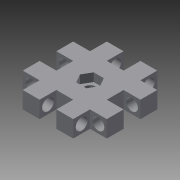
# Autodesk Inventor part: crossCenterMini
Saved by Autodesk Inventor 2015 (Build 190159000, 159)
## iProperties
Created: 2016-10-15
Part Number: crossCenterMini
Material: Generic
Document SubType Name: Modeling
Designer: Bardo91
Density: 1 g/cm^3
Appearance: Default
Author: Bardo91
Autodesk Inventor part; units mm, degrees
ref_plane "YZ Plane" through (0, 0, 0) normal (1, 0, 0) x (0, 1, 0)
ref_plane "XZ Plane" through (0, 0, 0) normal (0, 1, 0) x (-1, 0, 0)
ref_plane "XY Plane" through (0, 0, 0) normal (0, 0, 1) x (1, 0, 0)
sketch "Sketch1" plane through (0, 0, 0) normal (0, 0, 1) x (1, 0, 0)
  line L0 (0, 0) -> (0, 5)
  line L1 (0, 5) -> (5, 5)
  line L2 (5, 5) -> (5, 0)
  line L3 (5, 0) -> (10, 0)
  line L4 (10, 0) -> (10, 5)
  line L5 (10, 5) -> (15, 5)
  line L6 (15, 5) -> (15, 0)
  line L7 (15, 0) -> (20, 0)
  line L8 (20, 0) -> (20, -5)
  line L9 (20, -5) -> (15, -5)
  line L10 (15, -5) -> (15, -10)
  line L11 (15, -10) -> (20, -10)
  line L12 (20, -10) -> (20, -15)
  line L13 (20, -15) -> (15, -15)
  line L14 (15, -15) -> (15, -20)
  line L15 (15, -20) -> (10, -20)
  line L16 (10, -20) -> (10, -15)
  line L17 (10, -15) -> (5, -15)
  line L18 (5, -15) -> (5, -20)
  line L19 (5, -20) -> (0, -20)
  line L20 (0, -20) -> (0, -15)
  line L21 (0, -15) -> (-5, -15)
  line L22 (-5, -15) -> (-5, -10)
  line L23 (-5, -10) -> (0, -10)
  line L24 (0, -10) -> (0, -5)
  line L25 (0, -5) -> (-5, -5)
  line L26 (-5, -5) -> (-5, 0)
  line L27 (-5, 0) -> (0, 0)
  dimension "d0" = 5
  dimension "d1" = 5
  dimension "d2" = 5
  dimension "d3" = 5
  dimension "d4" = 5
  dimension "d5" = 5
  dimension "d6" = 5
  dimension "d7" = 5
  dimension "d8" = 5
  dimension "d9" = 5
  dimension "d10" = 5
  dimension "d11" = 5
  dimension "d12" = 5
  dimension "d13" = 5
  dimension "d14" = 5
  dimension "d15" = 5
  dimension "d16" = 5
  dimension "d17" = 5
  dimension "d18" = 5
  dimension "d19" = 5
  dimension "d20" = 5
  dimension "d21" = 5
  dimension "d22" = 5
  dimension "d23" = 5
  dimension "d24" = 5
  dimension "d25" = 90
  dimension "d26" = 5
  dimension "d27" = 5
  constraints: 56 end point, 16 point on line, 10 perpendicular, 2 vertical
  measures "d0" distance of L0.start L0.end
  measures "d1" distance of L0.end L1.end
  measures "d2" distance of L1.end L2.end
  measures "d3" distance of L2.end L3.end
  measures "d4" distance of L3.end L4.end
  measures "d5" distance of L4.end L5.end
  measures "d6" distance of L5.end L6.end
  measures "d7" distance of L6.end L7.end
  measures "d8" distance of L7.end L8.end
  measures "d9" distance of L8.end L9.end
  measures "d10" distance of L9.end L10.end
  measures "d11" distance of L10.end L11.end
  measures "d12" distance of L11.end L12.end
  measures "d13" distance of L12.end L13.end
  measures "d14" distance of L13.end L14.end
  measures "d15" distance of L14.end L15.end
  measures "d16" distance of L15.end L16.end
  measures "d17" distance of L16.end L17.end
  measures "d18" distance of L17.end L18.end
  measures "d19" distance of L18.end L19.end
  measures "d20" distance of L19.end L20.end
  measures "d21" distance of L20.end L21.end
  measures "d22" distance of L21.end L22.end
  measures "d23" distance of L22.end L23.end
  measures "d24" distance of L23.end L24.end
  measures "d25" angle of L24 L23
  measures "d26" distance of L24.end L25.end
  measures "d27" distance of L25.end L26.end
extrude "Extrusion1" add sketch "Sketch1" along normal blind 5
sketch "Sketch2" plane through (0, 0, 5) normal (0, 0, 1) x (1, 0, 0)
  line L0 (15, -10) -> (15, -5) projected
  line L1 (15, -7.5) -> (0, -7.5)
  line L2 (0, -10) -> (0, -5) projected
  circle A0 centre (7.5, -7.5) radius 1.75
  point P0 (0, 0)
  dimension "d30" = 3.5
  constraints: 3 midpoint, 2 end point, 1 centre point
  measures "d30" diameter of A0
extrude "Extrusion2" cut sketch "Sketch2" against normal blind 5
sketch "Sketch3" plane through (0, 0, 5) normal (0, 0, 1) x (1, 0, 0)
  circle A0 centre (7.5, -7.5) radius 1.75 projected
  line L0 (7.5, -7.5) -> (10.5, -7.5)
  line L1 (10.5, -7.5) -> (9, -4.9019)
  line L2 (7.5, -7.5) -> (9, -4.9019)
  point P0 (0, 0)
  dimension "d33" = 3
  dimension "d34" = 3
  dimension "d35" = 60
  constraints: 6 end point, 1 horizontal
  measures "d33" distance of L0.start L0.end
  measures "d34" distance of L0.end L1.end
  measures "d35" angle of L1 L0
extrude "Extrusion3" cut sketch "Sketch3" against normal blind 2.5 contours L0 L2 A0 | A0 L2 L1 L0 picked at (8.3623, -6.7236)
pattern_circular "Circular Pattern1" count 6 over 360 about axis through (7.5, -7.5, 5) along (0, 0, -1) of "Extrusion3"
sketch "Sketch4" plane through (-5, -15, 0) normal (0, -1, 0) x (1, 0, 0)
  line L0 (0, 5) -> (2.5, 5)
  line L1 (0, 5) -> (5, 5) projected
  line L2 (2.5, 5) -> (2.5, 2.5)
  circle A0 centre (2.5, 2.5) radius 1.75
  point P0 (5, 0)
  dimension "d41" = 2.5
  dimension "d42" = 2.5
  dimension "d43" = 3.5
  constraints: 4 end point, 1 centre point, 1 coincident, 1 midpoint, 1 perpendicular
  measures "d41" distance of L0.start L0.end
  measures "d42" distance of L0.end L2.end
  measures "d43" diameter of A0
extrude "Extrusion4" cut sketch "Sketch4" against normal through all
pattern_circular "Circular Pattern2" count 4 over 360 about axis through (7.5, -7.5, 5) along (0, 0, -1) of "Extrusion4"
body "Solid1"
